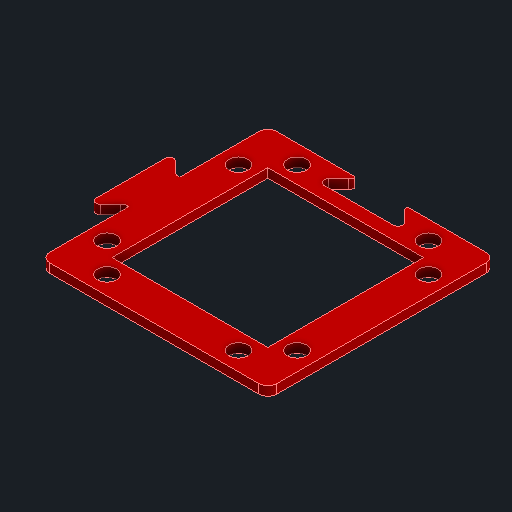
# Autodesk Inventor part: Interlinking Baseplate Pathed Angle V2
Saved by Autodesk Inventor 2023.4 (Build 274418000, 418)
## iProperties
Created: 2024-07-23
Part Number: Interlinking Baseplate Pathed Angle V2
Material: Generic
Document SubType Name: Modeling
Designer: xSibe
Density: 1 g/cm^3
Appearance: Plastic Dark Red
Author: xSibe
Autodesk Inventor part; units mm, degrees
ref_plane "YZ Plane" through (0, 0, 0) normal (1, 0, 0) x (0, 1, 0)
ref_plane "XZ Plane" through (0, 0, 0) normal (0, 1, 0) x (-1, 0, 0)
ref_plane "XY Plane" through (0, 0, 0) normal (0, 0, 1) x (1, 0, 0)
sketch "Sketch1" plane through (0, 0, 0) normal (0, 1, 0) x (-1, 0, 0)
  circle A0 centre (-21.9, -21.9) radius 1.875 projected
  circle A1 centre (21.9, 21.9) radius 1.875 projected
  circle A2 centre (21.9, -21.9) radius 1.875 projected
  circle A3 centre (-21.9, 21.9) radius 1.875 projected
  circle A4 centre (14.4, 20.8) radius 2.0734 projected
  circle A5 centre (-14.4, -20.8) radius 2.0734 projected
  circle A6 centre (14.4, -20.8) radius 2.0734 projected
  circle A7 centre (20.8, -14.4) radius 2.0734 projected
  line L0 (-17.05, 17.05) -> (-17.05, -17.05) projected
  line L1 (17.05, 17.05) -> (-17.05, 17.05) projected
  line L2 (17.05, -17.05) -> (17.05, 17.05) projected
  line L3 (-17.05, -17.05) -> (17.05, -17.05) projected
  circle A8 centre (20.8, 14.4) radius 2.0734 projected
  circle A9 centre (-14.4, 20.8) radius 2.0734 projected
  circle A10 centre (-20.8, -14.4) radius 2.0734 projected
  circle A11 centre (-20.8, 14.4) radius 2.0734 projected
  line L4 (-22.9, 24.875) -> (22.9, 24.875) projected
  arc A12 (-22.9, 24.875) -> (-24.875, 22.9) centre (-22.9, 22.9) ccw projected
  line L5 (-24.875, -22.9) -> (-24.875, 22.9) projected
  arc A13 (-24.875, -22.9) -> (-22.9, -24.875) centre (-22.9, -22.9) ccw projected
  line L6 (22.9, -24.875) -> (-22.9, -24.875) projected
  arc A14 (22.9, -24.875) -> (24.875, -22.9) centre (22.9, -22.9) ccw projected
  line L7 (24.875, 22.9) -> (24.875, -22.9) projected
  arc A15 (24.875, 22.9) -> (22.9, 24.875) centre (22.9, 22.9) ccw projected
  arc A16 (24.9, 22.9) -> (22.9, 24.9) centre (22.9, 22.9) ccw projected
  line L8 (22.9, 24.9) -> (-22.9, 24.9) projected
  arc A17 (-22.9, 24.9) -> (-24.9, 22.9) centre (-22.9, 22.9) ccw projected
  line L9 (-24.9, 22.9) -> (-24.9, -22.9) projected
  arc A18 (-24.9, -22.9) -> (-22.9, -24.9) centre (-22.9, -22.9) ccw projected
  line L10 (-22.9, -24.9) -> (22.9, -24.9) projected
  arc A19 (22.9, -24.9) -> (24.9, -22.9) centre (22.9, -22.9) ccw projected
  line L11 (24.9, -22.9) -> (24.9, 22.9) projected
  point P0 (0, 0)
extrude "Extrusion1" add sketch "Sketch1" along normal blind 2 contours A0 | A1 | A2 | A3 | L4 A15 L7 A14 L6 A13 L5 A12
sketch "Sketch2" plane through (0, 0, 0) normal (0, 1, 0) x (-1, 0, 0)
  line L0 (-7.5858, -29.875) -> (7.5858, -29.875)
  line L1 (10, -29.875) -> (10, -19.875)
  line L2 (7.5858, -19.875) -> (-7.5858, -19.875)
  line L3 (-10, -19.875) -> (-10, -29.875)
  line L4 (-10, -29.875) -> (10, -19.875) construction
  line L5 (10, -29.875) -> (-10, -19.875) construction
  line L6 (-8.2929, -21.5821) -> (-6.0607, -23.8143)
  line L7 (-10, -19.875) -> (-6.8431, -19.875) construction
  line L8 (8.2929, -21.5821) -> (6.0607, -23.8143)
  line L9 (-8.2929, -28.1679) -> (-6.0607, -25.9357)
  line L10 (8.2929, -28.1679) -> (6.0607, -25.9357)
  arc A0 (-8.2929, -28.1679) -> (-7.5858, -29.875) centre (-7.5858, -28.875) ccw
  arc A1 (7.5858, -29.875) -> (8.2929, -28.1679) centre (7.5858, -28.875) ccw
  arc A2 (-6.0607, -25.9357) -> (-6.0607, -23.8143) centre (-7.1213, -24.875) ccw
  arc A3 (6.0607, -23.8143) -> (6.0607, -25.9357) centre (7.1213, -24.875) ccw
  arc A4 (-7.5858, -19.875) -> (-8.2929, -21.5821) centre (-7.5858, -20.875) ccw
  arc A5 (8.2929, -21.5821) -> (7.5858, -19.875) centre (7.5858, -20.875) ccw
  line L11 (-7.5858, -19.95) -> (7.5858, -19.95)
  arc A6 (8.2399, -21.5291) -> (7.5858, -19.95) centre (7.5858, -20.875) ccw
  line L12 (8.2399, -21.5291) -> (6.0076, -23.7613)
  arc A7 (6.0076, -23.7613) -> (6.0076, -25.9887) centre (7.1213, -24.875) ccw
  line L13 (6.0076, -25.9887) -> (8.2399, -28.2209)
  arc A8 (7.5858, -29.8) -> (8.2399, -28.2209) centre (7.5858, -28.875) ccw
  line L14 (7.5858, -29.8) -> (-7.5858, -29.8)
  arc A9 (-8.2399, -28.2209) -> (-7.5858, -29.8) centre (-7.5858, -28.875) ccw
  line L15 (-8.2399, -28.2209) -> (-6.0076, -25.9887)
  arc A10 (-6.0076, -25.9887) -> (-6.0076, -23.7613) centre (-7.1213, -24.875) ccw
  line L16 (-6.0076, -23.7613) -> (-8.2399, -21.5291)
  arc A11 (-7.5858, -19.95) -> (-8.2399, -21.5291) centre (-7.5858, -20.875) ccw
  line L17 (-8.2399, 21.7791) -> (-6.0076, 24.0113)
  line L18 (-7.5858, 30.05) -> (7.5858, 30.05)
  line L19 (7.5858, 20.2) -> (-7.5858, 20.2)
  line L20 (-7.5858, 20.125) -> (7.5858, 20.125)
  line L21 (7.5858, 30.125) -> (-7.5858, 30.125)
  line L22 (10, 20.125) -> (-10, 30.125) construction
  line L23 (-10, 20.125) -> (10, 30.125) construction
  arc A12 (-6.0076, 24.0113) -> (-6.0076, 26.2387) centre (-7.1213, 25.125) ccw
  arc A13 (-6.0607, 24.0643) -> (-6.0607, 26.1857) centre (-7.1213, 25.125) ccw
  arc A14 (-7.5858, 30.05) -> (-8.2399, 28.4709) centre (-7.5858, 29.125) ccw
  arc A15 (-7.5858, 30.125) -> (-8.2929, 28.4179) centre (-7.5858, 29.125) ccw
  line L24 (-8.2929, 28.4179) -> (-6.0607, 26.1857)
  line L25 (-10, 30.125) -> (-6.8431, 30.125) construction
  line L26 (-10, 30.125) -> (-10, 20.125)
  arc A16 (-8.2399, 21.7791) -> (-7.5858, 20.2) centre (-7.5858, 21.125) ccw
  arc A17 (-8.2929, 21.8321) -> (-7.5858, 20.125) centre (-7.5858, 21.125) ccw
  line L27 (-8.2929, 21.8321) -> (-6.0607, 24.0643)
  line L28 (-6.0076, 26.2387) -> (-8.2399, 28.4709)
  line L29 (10, 20.125) -> (10, 30.125)
  line L30 (8.2929, 28.4179) -> (6.0607, 26.1857)
  line L31 (8.2929, 21.8321) -> (6.0607, 24.0643)
  arc A18 (7.5858, 20.125) -> (8.2929, 21.8321) centre (7.5858, 21.125) ccw
  arc A19 (6.0076, 26.2387) -> (6.0076, 24.0113) centre (7.1213, 25.125) ccw
  arc A20 (6.0607, 26.1857) -> (6.0607, 24.0643) centre (7.1213, 25.125) ccw
  arc A21 (7.5858, 20.2) -> (8.2399, 21.7791) centre (7.5858, 21.125) ccw
  line L32 (6.0076, 24.0113) -> (8.2399, 21.7791)
  line L33 (8.2399, 28.4709) -> (6.0076, 26.2387)
  arc A22 (8.2929, 28.4179) -> (7.5858, 30.125) centre (7.5858, 29.125) ccw
  arc A23 (8.2399, 28.4709) -> (7.5858, 30.05) centre (7.5858, 29.125) ccw
  line L34 (0, 24.875) -> (0, 25.125)
  line L35 (-22.9, -24.875) -> (22.9, -24.875) projected
  line L36 (22.9, 24.875) -> (-22.9, 24.875) projected
  line L37 (0, -24.875) -> (0, -24.875)
  line L38 (5.6213, 25.125) -> (5.5463, 25.125)
  line L39 (5.5463, 25.125) -> (5.5463, 24.875)
  line L40 (5.5463, 24.875) -> (5.6213, 24.875)
  line L41 (5.6213, 24.875) -> (5.6213, 25.125)
  line L42 (-5.6213, 25.125) -> (-5.5463, 25.125)
  line L43 (-5.5463, 25.125) -> (-5.5463, 24.875)
  line L44 (-5.5463, 24.875) -> (-5.6213, 24.875)
  line L45 (-5.6213, 24.875) -> (-5.6213, 25.125)
  line L46 (-5.6213, -24.875) -> (-5.5463, -24.875)
  line L47 (-5.5463, -24.875) -> (-5.5463, -24.875)
  line L48 (-5.5463, -24.875) -> (-5.6213, -24.875)
  line L49 (-5.6213, -24.875) -> (-5.6213, -24.875)
  line L50 (5.6213, -24.875) -> (5.5463, -24.875)
  line L51 (5.5463, -24.875) -> (5.5463, -24.875)
  line L52 (5.5463, -24.875) -> (5.6213, -24.875)
  line L53 (5.6213, -24.875) -> (5.6213, -24.875)
  arc A24 (19.95, -7.5858) -> (21.5291, -8.2399) centre (20.875, -7.5858) ccw
  arc A25 (19.875, -7.5858) -> (21.5821, -8.2929) centre (20.875, -7.5858) ccw
  line L54 (21.5821, -8.2929) -> (23.8143, -6.0607)
  line L55 (23.7613, -6.0076) -> (21.5291, -8.2399)
  arc A26 (25.9357, -6.0607) -> (23.8143, -6.0607) centre (24.875, -7.1213) ccw
  arc A27 (25.9887, -6.0076) -> (23.7613, -6.0076) centre (24.875, -7.1213) ccw
  line L56 (29.875, -7.5858) -> (29.875, 7.5858)
  line L57 (29.8, 7.5858) -> (29.8, -7.5858)
  line L58 (19.95, -7.5858) -> (19.95, 7.5858)
  line L59 (19.875, 7.5858) -> (19.875, -7.5858)
  line L60 (28.2209, -8.2399) -> (25.9887, -6.0076)
  line L61 (21.5821, 8.2929) -> (23.8143, 6.0607)
  line L62 (28.1679, 8.2929) -> (25.9357, 6.0607)
  arc A28 (29.875, 7.5858) -> (28.1679, 8.2929) centre (28.875, 7.5858) ccw
  arc A29 (23.7613, 6.0076) -> (25.9887, 6.0076) centre (24.875, 7.1213) ccw
  line L63 (24.875, 5.5463) -> (24.875, 5.5463)
  line L64 (24.875, 5.6213) -> (24.875, 5.5463)
  line L65 (24.875, 5.5463) -> (24.875, 5.6213)
  line L66 (24.875, 5.6213) -> (24.875, 5.6213)
  arc A30 (23.8143, 6.0607) -> (25.9357, 6.0607) centre (24.875, 7.1213) ccw
  line L67 (25.9887, 6.0076) -> (28.2209, 8.2399)
  arc A31 (29.8, 7.5858) -> (28.2209, 8.2399) centre (28.875, 7.5858) ccw
  line L68 (21.5291, 8.2399) -> (23.7613, 6.0076)
  arc A32 (21.5291, 8.2399) -> (19.95, 7.5858) centre (20.875, 7.5858) ccw
  arc A33 (21.5821, 8.2929) -> (19.875, 7.5858) centre (20.875, 7.5858) ccw
  line L69 (24.875, -5.5463) -> (24.875, -5.5463)
  line L70 (24.875, -5.5463) -> (24.875, -5.6213)
  line L71 (24.875, -5.6213) -> (24.875, -5.5463)
  line L72 (24.875, -5.6213) -> (24.875, -5.6213)
  line L73 (24.875, 0) -> (24.875, 0)
  line L74 (28.1679, -8.2929) -> (25.9357, -6.0607)
  arc A34 (28.1679, -8.2929) -> (29.875, -7.5858) centre (28.875, -7.5858) ccw
  arc A35 (28.2209, -8.2399) -> (29.8, -7.5858) centre (28.875, -7.5858) ccw
  line L75 (-25.125, 5.6213) -> (-25.125, 5.5463)
  arc A36 (-28.4709, 8.2399) -> (-30.05, 7.5858) centre (-29.125, 7.5858) ccw
  arc A37 (-28.4179, 8.2929) -> (-30.125, 7.5858) centre (-29.125, 7.5858) ccw
  line L76 (-28.4179, 8.2929) -> (-26.1857, 6.0607)
  line L77 (-24.875, 5.5463) -> (-24.875, 5.6213)
  arc A38 (-26.2387, 6.0076) -> (-24.0113, 6.0076) centre (-25.125, 7.1213) ccw
  line L78 (-21.8321, 8.2929) -> (-24.0643, 6.0607)
  line L79 (-24.875, 0) -> (-25.125, 0)
  arc A39 (-20.2, 7.5858) -> (-21.7791, 8.2399) centre (-21.125, 7.5858) ccw
  arc A40 (-20.125, 7.5858) -> (-21.8321, 8.2929) centre (-21.125, 7.5858) ccw
  line L80 (-30.05, -7.5858) -> (-30.05, 7.5858)
  line L81 (-30.125, 7.5858) -> (-30.125, -7.5858)
  line L82 (-20.2, 7.5858) -> (-20.2, -7.5858)
  line L83 (-20.125, -7.5858) -> (-20.125, 7.5858)
  line L84 (-24.875, 5.6213) -> (-25.125, 5.6213)
  arc A41 (-26.1857, 6.0607) -> (-24.0643, 6.0607) centre (-25.125, 7.1213) ccw
  line L85 (-24.0113, 6.0076) -> (-21.7791, 8.2399)
  line L86 (-25.125, 5.5463) -> (-24.875, 5.5463)
  line L87 (-28.4709, 8.2399) -> (-26.2387, 6.0076)
  line L88 (-25.125, -5.5463) -> (-24.875, -5.5463)
  line L89 (-24.875, -5.5463) -> (-24.875, -5.6213)
  line L90 (-24.875, -5.6213) -> (-25.125, -5.6213)
  line L91 (-25.125, -5.6213) -> (-25.125, -5.5463)
  arc A42 (-30.05, -7.5858) -> (-28.4709, -8.2399) centre (-29.125, -7.5858) ccw
  arc A43 (-21.8321, -8.2929) -> (-20.125, -7.5858) centre (-21.125, -7.5858) ccw
  arc A44 (-21.7791, -8.2399) -> (-20.2, -7.5858) centre (-21.125, -7.5858) ccw
  arc A45 (-24.0113, -6.0076) -> (-26.2387, -6.0076) centre (-25.125, -7.1213) ccw
  arc A46 (-24.0643, -6.0607) -> (-26.1857, -6.0607) centre (-25.125, -7.1213) ccw
  line L92 (-21.7791, -8.2399) -> (-24.0113, -6.0076)
  line L93 (-21.8321, -8.2929) -> (-24.0643, -6.0607)
  line L94 (-28.4179, -8.2929) -> (-26.1857, -6.0607)
  line L95 (-26.2387, -6.0076) -> (-28.4709, -8.2399)
  arc A47 (-30.125, -7.5858) -> (-28.4179, -8.2929) centre (-29.125, -7.5858) ccw
  arc A48 (7.5858, 19.95) -> (8.2399, 21.5291) centre (7.5858, 20.875) ccw
  arc A49 (7.5858, 19.875) -> (8.2929, 21.5821) centre (7.5858, 20.875) ccw
  line L96 (8.2929, 21.5821) -> (6.0607, 23.8143)
  line L97 (6.0076, 23.7613) -> (8.2399, 21.5291)
  arc A50 (6.0607, 25.9357) -> (6.0607, 23.8143) centre (7.1213, 24.875) ccw
  arc A51 (6.0076, 25.9887) -> (6.0076, 23.7613) centre (7.1213, 24.875) ccw
  line L98 (7.5858, 29.875) -> (-7.5858, 29.875)
  line L99 (-7.5858, 29.8) -> (7.5858, 29.8)
  line L100 (7.5858, 19.95) -> (-7.5858, 19.95)
  line L101 (-7.5858, 19.875) -> (7.5858, 19.875)
  line L102 (8.2399, 28.2209) -> (6.0076, 25.9887)
  line L103 (-8.2929, 21.5821) -> (-6.0607, 23.8143)
  line L104 (-8.2929, 28.1679) -> (-6.0607, 25.9357)
  arc A52 (-7.5858, 29.875) -> (-8.2929, 28.1679) centre (-7.5858, 28.875) ccw
  arc A53 (-6.0076, 23.7613) -> (-6.0076, 25.9887) centre (-7.1213, 24.875) ccw
  line L105 (-5.5463, 24.875) -> (-5.5463, 24.875)
  line L106 (-5.6213, 24.875) -> (-5.5463, 24.875)
  line L107 (-5.5463, 24.875) -> (-5.6213, 24.875)
  line L108 (-5.6213, 24.875) -> (-5.6213, 24.875)
  arc A54 (-6.0607, 23.8143) -> (-6.0607, 25.9357) centre (-7.1213, 24.875) ccw
  line L109 (-6.0076, 25.9887) -> (-8.2399, 28.2209)
  arc A55 (-7.5858, 29.8) -> (-8.2399, 28.2209) centre (-7.5858, 28.875) ccw
  line L110 (-8.2399, 21.5291) -> (-6.0076, 23.7613)
  arc A56 (-8.2399, 21.5291) -> (-7.5858, 19.95) centre (-7.5858, 20.875) ccw
  arc A57 (-8.2929, 21.5821) -> (-7.5858, 19.875) centre (-7.5858, 20.875) ccw
  line L111 (5.5463, 24.875) -> (5.5463, 24.875)
  line L112 (5.5463, 24.875) -> (5.6213, 24.875)
  line L113 (5.6213, 24.875) -> (5.5463, 24.875)
  line L114 (5.6213, 24.875) -> (5.6213, 24.875)
  line L115 (0, 24.875) -> (0, 24.875)
  line L116 (8.2929, 28.1679) -> (6.0607, 25.9357)
  arc A58 (8.2929, 28.1679) -> (7.5858, 29.875) centre (7.5858, 28.875) ccw
  arc A59 (8.2399, 28.2209) -> (7.5858, 29.8) centre (7.5858, 28.875) ccw
  line L117 (-5.6213, -25.125) -> (-5.5463, -25.125)
  arc A60 (-8.2399, -28.4709) -> (-7.5858, -30.05) centre (-7.5858, -29.125) ccw
  arc A61 (-8.2929, -28.4179) -> (-7.5858, -30.125) centre (-7.5858, -29.125) ccw
  line L118 (-8.2929, -28.4179) -> (-6.0607, -26.1857)
  line L119 (-5.5463, -24.875) -> (-5.6213, -24.875)
  arc A62 (-6.0076, -26.2387) -> (-6.0076, -24.0113) centre (-7.1213, -25.125) ccw
  line L120 (-8.2929, -21.8321) -> (-6.0607, -24.0643)
  line L121 (0, -24.875) -> (0, -25.125)
  arc A63 (-7.5858, -20.2) -> (-8.2399, -21.7791) centre (-7.5858, -21.125) ccw
  arc A64 (-7.5858, -20.125) -> (-8.2929, -21.8321) centre (-7.5858, -21.125) ccw
  line L122 (7.5858, -30.05) -> (-7.5858, -30.05)
  line L123 (-7.5858, -30.125) -> (7.5858, -30.125)
  line L124 (-7.5858, -20.2) -> (7.5858, -20.2)
  line L125 (7.5858, -20.125) -> (-7.5858, -20.125)
  line L126 (-5.6213, -24.875) -> (-5.6213, -25.125)
  arc A65 (-6.0607, -26.1857) -> (-6.0607, -24.0643) centre (-7.1213, -25.125) ccw
  line L127 (-6.0076, -24.0113) -> (-8.2399, -21.7791)
  line L128 (-5.5463, -25.125) -> (-5.5463, -24.875)
  line L129 (-8.2399, -28.4709) -> (-6.0076, -26.2387)
  line L130 (5.5463, -25.125) -> (5.5463, -24.875)
  line L131 (5.5463, -24.875) -> (5.6213, -24.875)
  line L132 (5.6213, -24.875) -> (5.6213, -25.125)
  line L133 (5.6213, -25.125) -> (5.5463, -25.125)
  arc A66 (7.5858, -30.05) -> (8.2399, -28.4709) centre (7.5858, -29.125) ccw
  arc A67 (8.2929, -21.8321) -> (7.5858, -20.125) centre (7.5858, -21.125) ccw
  arc A68 (8.2399, -21.7791) -> (7.5858, -20.2) centre (7.5858, -21.125) ccw
  arc A69 (6.0076, -24.0113) -> (6.0076, -26.2387) centre (7.1213, -25.125) ccw
  arc A70 (6.0607, -24.0643) -> (6.0607, -26.1857) centre (7.1213, -25.125) ccw
  line L134 (8.2399, -21.7791) -> (6.0076, -24.0113)
  line L135 (8.2929, -21.8321) -> (6.0607, -24.0643)
  line L136 (8.2929, -28.4179) -> (6.0607, -26.1857)
  line L137 (6.0076, -26.2387) -> (8.2399, -28.4709)
  arc A71 (7.5858, -30.125) -> (8.2929, -28.4179) centre (7.5858, -29.125) ccw
  arc A72 (-19.95, 7.5858) -> (-21.5291, 8.2399) centre (-20.875, 7.5858) ccw
  arc A73 (-19.875, 7.5858) -> (-21.5821, 8.2929) centre (-20.875, 7.5858) ccw
  line L138 (-21.5821, 8.2929) -> (-23.8143, 6.0607)
  line L139 (-23.7613, 6.0076) -> (-21.5291, 8.2399)
  arc A74 (-25.9357, 6.0607) -> (-23.8143, 6.0607) centre (-24.875, 7.1213) ccw
  arc A75 (-25.9887, 6.0076) -> (-23.7613, 6.0076) centre (-24.875, 7.1213) ccw
  line L140 (-29.875, 7.5858) -> (-29.875, -7.5858)
  line L141 (-29.8, -7.5858) -> (-29.8, 7.5858)
  line L142 (-19.95, 7.5858) -> (-19.95, -7.5858)
  line L143 (-19.875, -7.5858) -> (-19.875, 7.5858)
  line L144 (-28.2209, 8.2399) -> (-25.9887, 6.0076)
  line L145 (-21.5821, -8.2929) -> (-23.8143, -6.0607)
  line L146 (-28.1679, -8.2929) -> (-25.9357, -6.0607)
  arc A76 (-29.875, -7.5858) -> (-28.1679, -8.2929) centre (-28.875, -7.5858) ccw
  arc A77 (-23.7613, -6.0076) -> (-25.9887, -6.0076) centre (-24.875, -7.1213) ccw
  line L147 (-24.875, -5.5463) -> (-24.875, -5.5463)
  line L148 (-24.875, -5.6213) -> (-24.875, -5.5463)
  line L149 (-24.875, -5.5463) -> (-24.875, -5.6213)
  line L150 (-24.875, -5.6213) -> (-24.875, -5.6213)
  arc A78 (-23.8143, -6.0607) -> (-25.9357, -6.0607) centre (-24.875, -7.1213) ccw
  line L151 (-25.9887, -6.0076) -> (-28.2209, -8.2399)
  arc A79 (-29.8, -7.5858) -> (-28.2209, -8.2399) centre (-28.875, -7.5858) ccw
  line L152 (-21.5291, -8.2399) -> (-23.7613, -6.0076)
  arc A80 (-21.5291, -8.2399) -> (-19.95, -7.5858) centre (-20.875, -7.5858) ccw
  arc A81 (-21.5821, -8.2929) -> (-19.875, -7.5858) centre (-20.875, -7.5858) ccw
  line L153 (-24.875, 5.5463) -> (-24.875, 5.5463)
  line L154 (-24.875, 5.5463) -> (-24.875, 5.6213)
  line L155 (-24.875, 5.6213) -> (-24.875, 5.5463)
  line L156 (-24.875, 5.6213) -> (-24.875, 5.6213)
  line L157 (-24.875, 0) -> (-24.875, 0)
  line L158 (-28.1679, 8.2929) -> (-25.9357, 6.0607)
  arc A82 (-28.1679, 8.2929) -> (-29.875, 7.5858) centre (-28.875, 7.5858) ccw
  arc A83 (-28.2209, 8.2399) -> (-29.8, 7.5858) centre (-28.875, 7.5858) ccw
  line L159 (25.125, -5.6213) -> (25.125, -5.5463)
  arc A84 (28.4709, -8.2399) -> (30.05, -7.5858) centre (29.125, -7.5858) ccw
  arc A85 (28.4179, -8.2929) -> (30.125, -7.5858) centre (29.125, -7.5858) ccw
  line L160 (28.4179, -8.2929) -> (26.1857, -6.0607)
  line L161 (24.875, -5.5463) -> (24.875, -5.6213)
  arc A86 (26.2387, -6.0076) -> (24.0113, -6.0076) centre (25.125, -7.1213) ccw
  line L162 (21.8321, -8.2929) -> (24.0643, -6.0607)
  line L163 (24.875, 0) -> (25.125, 0)
  arc A87 (20.2, -7.5858) -> (21.7791, -8.2399) centre (21.125, -7.5858) ccw
  arc A88 (20.125, -7.5858) -> (21.8321, -8.2929) centre (21.125, -7.5858) ccw
  line L164 (30.05, 7.5858) -> (30.05, -7.5858)
  line L165 (30.125, -7.5858) -> (30.125, 7.5858)
  line L166 (20.2, -7.5858) -> (20.2, 7.5858)
  line L167 (20.125, 7.5858) -> (20.125, -7.5858)
  line L168 (24.875, -5.6213) -> (25.125, -5.6213)
  arc A89 (26.1857, -6.0607) -> (24.0643, -6.0607) centre (25.125, -7.1213) ccw
  line L169 (24.0113, -6.0076) -> (21.7791, -8.2399)
  line L170 (25.125, -5.5463) -> (24.875, -5.5463)
  line L171 (28.4709, -8.2399) -> (26.2387, -6.0076)
  line L172 (25.125, 5.5463) -> (24.875, 5.5463)
  line L173 (24.875, 5.5463) -> (24.875, 5.6213)
  line L174 (24.875, 5.6213) -> (25.125, 5.6213)
  line L175 (25.125, 5.6213) -> (25.125, 5.5463)
  arc A90 (30.05, 7.5858) -> (28.4709, 8.2399) centre (29.125, 7.5858) ccw
  arc A91 (21.8321, 8.2929) -> (20.125, 7.5858) centre (21.125, 7.5858) ccw
  arc A92 (21.7791, 8.2399) -> (20.2, 7.5858) centre (21.125, 7.5858) ccw
  arc A93 (24.0113, 6.0076) -> (26.2387, 6.0076) centre (25.125, 7.1213) ccw
  arc A94 (24.0643, 6.0607) -> (26.1857, 6.0607) centre (25.125, 7.1213) ccw
  line L176 (21.7791, 8.2399) -> (24.0113, 6.0076)
  line L177 (21.8321, 8.2929) -> (24.0643, 6.0607)
  line L178 (28.4179, 8.2929) -> (26.1857, 6.0607)
  line L179 (26.2387, 6.0076) -> (28.4709, 8.2399)
  arc A95 (30.125, 7.5858) -> (28.4179, 8.2929) centre (29.125, 7.5858) ccw
  line L180 (-22.9, -24.875) -> (22.9, -24.875) projected
  arc A96 (22.9, -24.875) -> (24.875, -22.9) centre (22.9, -22.9) ccw projected
  line L181 (24.875, -22.9) -> (24.875, 22.9) projected
  arc A97 (24.875, 22.9) -> (22.9, 24.875) centre (22.9, 22.9) ccw projected
  line L182 (22.9, 24.875) -> (-22.9, 24.875) projected
  arc A98 (-22.9, 24.875) -> (-24.875, 22.9) centre (-22.9, 22.9) ccw projected
  line L183 (-24.875, 22.9) -> (-24.875, -22.9) projected
  arc A99 (-24.875, -22.9) -> (-22.9, -24.875) centre (-22.9, -22.9) ccw projected
  circle A100 centre (-20.8, 14.4) radius 2.0734 projected
  circle A101 centre (-20.8, -14.4) radius 2.0734 projected
  circle A102 centre (-14.4, 20.8) radius 2.0734 projected
  circle A103 centre (20.8, 14.4) radius 2.0734 projected
  circle A104 centre (20.8, -14.4) radius 2.0734 projected
  circle A105 centre (14.4, -20.8) radius 2.0734 projected
  circle A106 centre (-14.4, -20.8) radius 2.0734 projected
  circle A107 centre (14.4, 20.8) radius 2.0734 projected
  line L184 (-17.05, 17.05) -> (17.05, 17.05) projected
  line L185 (17.05, 17.05) -> (17.05, -17.05) projected
  line L186 (17.05, -17.05) -> (-17.05, -17.05) projected
  line L187 (-17.05, -17.05) -> (-17.05, 17.05) projected
  point P0 (0, 0)
  point P1 (19.875, -6.8431)
  point P2 (19.875, -10)
  point P3 (29.875, -10)
  point P4 (29.875, 10)
  point P5 (19.875, 10)
  point P6 (-30.125, 10)
  point P7 (-20.125, 10)
  point P8 (-30.125, -10)
  point P9 (-20.125, -10)
  point P10 (-30.125, -6.8431)
  point P11 (6.8431, 19.875)
  point P12 (10, 19.875)
  point P13 (10, 29.875)
  point P14 (-10, 29.875)
  point P15 (-10, 19.875)
  point P16 (-10, -30.125)
  point P17 (-10, -20.125)
  point P18 (10, -30.125)
  point P19 (10, -20.125)
  point P20 (6.8431, -30.125)
  point P21 (-19.875, 6.8431)
  point P22 (-19.875, 10)
  point P23 (-29.875, 10)
  point P24 (-29.875, -10)
  point P25 (-19.875, -10)
  point P26 (30.125, -10)
  point P27 (20.125, -10)
  point P28 (30.125, 10)
  point P29 (20.125, 10)
  point P30 (30.125, 6.8431)
  point P31 (-21, 8.5023)
  point P32 (-24.625, 5.5463)
  point P33 (-25.125, 5.5463)
  point P34 (-25.125, -5.5463)
  point P35 (-24.625, -5.5463)
  point P36 (-21, -8.5023)
  point P37 (-5.5463, 25.125)
  point P38 (5.5463, 25.125)
  dimension "d19" = 20
  dimension "d20" = 10
  dimension "d21" = 45
  dimension "d22" = 1
  dimension "d23" = 1.5
  dimension "d24" = 1
  dimension "d25" = 0.075
  dimension "d28" = 15.1716
  dimension "d29" = 2.8787
  dimension "d30" = 2.8787
  dimension "d31" = 20
  dimension "d32" = 10
  dimension "d33" = 45
  dimension "d34" = 1
  dimension "d35" = 1.5
  dimension "d36" = 1
  dimension "d37" = 0.075
  dimension "d38" = 15.1716
  dimension "d39" = 2.8787
  dimension "d40" = 2.8787
  dimension "d41" = 0.25
  dimension "d42" = 0
  dimension "d45" = 360
  constraints: 356 end point, 196 point on circle, 96 centre point, 68 point on line, 28 tangent, 16 equal length, 8 horizontal, 6 equal radius, 6 midpoint, 6 perpendicular, 2 vertical, 647 other
  measures "d19" distance of L5.end L4.end
  measures "d20" distance of L5.start L4.end
  measures "d21" angle of L6 L7
  measures "d22" radius of A0
  measures "d23" radius of A2
  measures "d24" radius of A4
  measures "d25" distance between parallel lines of L2 L11
  measures "d28" distance of A9.centre A1.centre
  measures "d29" distance from line of A7.centre L1
  measures "d30" distance from line of L3 A10.centre
  measures "d31" distance of L22.end L29.end
  measures "d32" distance of L29.start L29.end
  measures "d33" angle of L24 L25
  measures "d34" radius of A17
  measures "d35" radius of A13
  measures "d36" radius of A15
  measures "d37" distance between parallel lines of L21 L18
  measures "d38" distance of A16.centre A21.centre
  measures "d39" distance from line of A19.centre L29
  measures "d40" distance from line of L26 A12.centre
  measures "d41" distance of L34.start L34.end
  measures "d42" distance of L37.start L37.end
extrude "Extrusion2" add sketch "Sketch2" along normal up to surface (2 mm away) contours L181 L172 A93 L179 A90 A31 L57 A35 A84 L171 A86 L170 | A84 A35 L57 A31 A90 A28 L56 A34 | A34 L56 A28 A90 L164 A84
extrude "Extrusion3" cut sketch "Sketch2" along normal up to surface (2 mm away) contours A2 A62 L35 | L35 A62 A2 L6 A4 A63 A11 L16 A10 | A10 L16 A11 A63 L124 A68 A6 L12 A7 L35 | L35 A69 A3 | A7 L12 A6 A68 A5 L8 A3 A69 L35 | A64 A11 A63 A4 | A4 L2 A5 A67 A6 L11 A11 A64 | A11 A64 L125 A67 A6 A68 L124 A63 | A5 A68 A6 A67 | A11 L11 A6 A67 L125 A64
fillet "Fillet1" radius 0.25 2 edges at (5.6213, 1, -24.875) (-5.6213, 1, -24.875)
body "Solid1"
